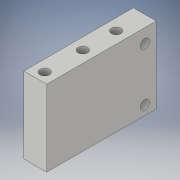
# Autodesk Inventor part: Motorhalterung_Grundplatte
Saved by Autodesk Inventor 2018 (Build 220112000, 112)
## iProperties
Created: 2018-03-26
Part Number: Motorhalterung_Grundplatte
Material: Generisch
Document SubType Name: Modeling
Designer: Julian
Density: 1 g/cm^3
Appearance: Vorgabe
Author: Julian
Autodesk Inventor part; units mm, degrees
ref_plane "YZ Plane" through (0, 0, 0) normal (1, 0, 0) x (0, 1, 0)
ref_plane "XZ Plane" through (0, 0, 0) normal (0, 1, 0) x (-1, 0, 0)
ref_plane "XY Plane" through (0, 0, 0) normal (0, 0, 1) x (1, 0, 0)
sketch "Skizze1" plane through (0, 0, 0) normal (0, 0, 1) x (1, 0, 0)
  line L0 (0, 0) -> (24, 0)
  line L1 (24, 0) -> (24, 115)
  line L2 (24, 115) -> (0, 115)
  line L3 (0, 115) -> (0, 0)
  dimension "d0" = 24
  dimension "d1" = 115
  constraints: 8 end point, 2 parallel, 1 horizontal, 1 perpendicular
  measures "d0" distance of L2.end L1.end
  measures "d1" distance of L1.end L0.end
extrude "Extrusion1" add sketch "Skizze1" along normal blind 80
sketch "Skizze2" plane through (0, 0, 0) normal (-1, 0, 0) x (0, 0, 1)
  line L0 (0, 0) -> (0, 115) projected
  line L1 (0, 115) -> (0, 103)
  line L2 (0, 103) -> (9.875, 103)
  line L3 (9.875, 103) -> (65.375, 103)
  dimension "d4" = 12
  dimension "d5" = 9.875
  dimension "d6" = 55.5
  constraints: 6 end point, 2 point on line, 1 horizontal
  measures "d4" distance of L0.end L1.end
  measures "d5" distance of L1.end L2.end
  measures "d6" distance of L2.end L3.end
hole "Bohrung1" at (0, 103, 9.875) at (0, 103, 65.375) direction (1, 0, 0) diameter 9.5 end through all
sketch "Skizze3" plane through (0, 0, 80) normal (0, 0, 1) x (1, 0, 0)
  line L0 (24, 115) -> (0, 115) projected
  line L1 (12, 115) -> (12, 85)
  line L2 (12, 85) -> (12, 50)
  line L3 (12, 50) -> (12, 10)
  point P0 (0, 0)
  dimension "d14" = 30
  dimension "d15" = 35
  dimension "d16" = 40
  constraints: 6 end point, 2 vertical, 1 midpoint, 1 point on line
  measures "d14" distance of L1.start L1.end
  measures "d15" distance of L1.end L2.end
  measures "d16" distance of L2.end L3.end
hole "Bohrung2" at (12, 85, 80) at (12, 10, 80) at (12, 50, 80) direction (0, 0, -1) diameter 10 end through all
